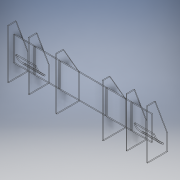
# Autodesk Inventor part: F-wing
Saved by Autodesk Inventor 2018.1 (Build 221171000, 171)
## iProperties
Created: 2017-10-11
Part Number: F-wing
Material: 一般
Document SubType Name: Modeling
Designer: kuwano
Density: 1 g/cm^3
Appearance: 既定
Author: kuwano
Autodesk Inventor part; units mm, degrees
sketch "スケッチ1" plane through (0, 0, 0) normal (1, 0, 0) x (0, 1, 0)
  line L0 (10, 125) -> (0, 125)
  line L1 (0, 125) -> (0, -125)
  line L2 (0, -125) -> (10, -125)
  line L3 (10, -125) -> (10, 125)
  point P0 (0, 0)
  dimension "d0" = 250
  dimension "d1" = 10
  constraints: 8 end point, 2 midpoint, 2 parallel, 1 horizontal, 1 perpendicular
  measures "d0" distance of L0.end L1.end
  measures "d1" distance of L1.end L2.end
extrude "押し出し1" add sketch "スケッチ1" along normal mid plane 1400
sketch "スケッチ2" plane through (700, 0, 0) normal (1, 0, 0) x (0, 0, -1)
  line L0 (104.6973, 150) -> (-225, 30)
  line L1 (-225, 30) -> (-225, -50)
  line L2 (-225, -50) -> (275, -50)
  line L3 (275, -50) -> (275, 150)
  line L4 (-125, 0) -> (125, 0) projected
  line L5 (-125, 10) -> (-125, 0) projected
  line L6 (125, 0) -> (125, 10) projected
  line L7 (125, 10) -> (-125, 10) projected
  line L8 (104.6973, 150) -> (275, 150)
  point P0 (0, 0)
  dimension "d4" = 50
  dimension "d5" = 20
  dimension "d6" = 200
  dimension "d7" = 500
  dimension "d8" = 100
  dimension "d9" = 80
  constraints: 10 end point, 3 parallel, 1 horizontal
  measures "d4" distance between parallel lines of L2 L4
  measures "d5" angle of L7 L0
  measures "d6" distance of L2.end L3.end
  measures "d7" distance of L1.end L2.end
  measures "d8" distance between parallel lines of L5 L1
  measures "d9" distance of L0.end L1.end
extrude "押し出し3" add sketch "スケッチ2" along normal blind 10 contours L8 L3 L2 L1 L0 | L5 L7 L6 L4
ref_plane "作業平面1" through (230, 0, 0) normal (1, 0, 0) x (0, 1, 0)
ref_plane "作業平面2" through (600, 0, 0) normal (-1, 0, 0) x (0, 0, 1)
ref_plane "作業平面3" through (230, 0, 0) normal (1, 0, 0) x (0, 1, 0)
mirror "ミラー3" about plane through (600, 0, 0) normal (-1, 0, 0) of "押し出し3"
sketch "スケッチ4" plane through (230, 0, 0) normal (1, 0, 0) x (0, 1, 0)
  line L0 (40, 205) -> (-30, 205)
  line L1 (-30, 205) -> (-30, -325)
  line L2 (-30, -325) -> (200, -325)
  line L3 (200, -325) -> (200, -72.1281)
  line L4 (200, -72.1281) -> (40, 205)
  line L5 (0, -520.2563) -> (0, 349.2094) projected
  line L6 (30, 225) -> (-50, 225) projected
  line L7 (-50, 225) -> (-50, -275) projected
  line L8 (-50, -275) -> (150, -275) projected
  point P0 (0, 0)
  dimension "d25" = 230
  dimension "d26" = 20
  dimension "d27" = 20
  dimension "d28" = 50
  dimension "d29" = 30
  dimension "d30" = 70
  constraints: 10 end point, 2 parallel, 1 horizontal, 1 perpendicular
  measures "d25" distance of L1.end L2.end
  measures "d26" distance between parallel lines of L6 L0
  measures "d27" distance between parallel lines of L7 L1
  measures "d28" distance between parallel lines of L2 L8
  measures "d29" angle of L1 L4
  measures "d30" distance of L0.start L0.end
extrude "押し出し5" add sketch "スケッチ4" along normal blind 10 contours L4 L3 L2 L5 L0 | L5 L8 L1 L0 | L5 L2 L1 L8
sketch "スケッチ5" plane through (700, 0, 0) normal (-1, 0, 0) x (0, 0, 1)
  arc A0 (-199.5342, 116.4458) -> (-65, 20) centre (4.9464, 259.6246) ccw
  arc A1 (-191.3426, 122.1816) -> (-62.1979, 29.5994) centre (4.9464, 259.6246) ccw
  line L0 (-65, 20) -> (-62.1979, 29.5994)
  line L1 (-191.3426, 122.1816) -> (-199.5342, 116.4458)
  line L2 (125, 10) -> (-125, 10) projected
  line L3 (-125, 10) -> (-125, 0) projected
  line L4 (-125, 10) -> (-199.5342, 116.4458)
  point P0 (0, 0)
  dimension "d33" = 10
  dimension "d36" = 10
  dimension "d37" = 60
  dimension "d42" = 125
  constraints: 6 end point, 4 point on circle, 2 centre point, 2 line through centre, 2 tangent, 1 concentric
  measures "d33" radial gap between concentric circles of A1 A0
  measures "d36" distance from line of L2 L0.start
  measures "d37" distance from line of L0.start L3
  measures "d42" angle of L2 L4
extrude "押し出し6" add sketch "スケッチ5" along normal up to next
mirror "ミラー5" about plane through (0, 0, 0) normal (1, 0, 0) of "押し出し5", "押し出し3", "ミラー3", "押し出し6"
